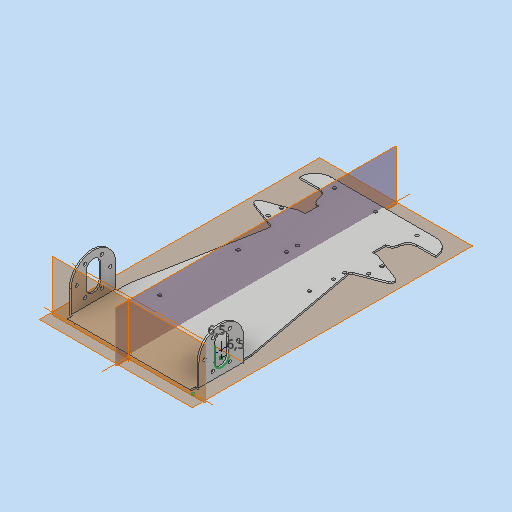
# Autodesk Inventor part: grundplatte
Saved by Autodesk Inventor 2022 (Build 260153000, 153)
## iProperties
Created: 2021-05-24
Part Number: grundplatte
Material: Generisch
Document SubType Name: Modeling
Designer: Lukas
Density: 1 g/cm^3
Appearance: Vorgabe
Author: Lukas
Autodesk Inventor part; units mm, degrees
sketch "Skizze1" plane through (0, 0, 0) normal (0, 1, 0) x (-1, 0, 0)
  line L0 (-55, 0) -> (-55, -55)
  line L1 (-55, -55) -> (-35.3027, -161.5294)
  line L2 (0, 0) -> (-55, 0)
  line L3 (79.5383, 0) -> (-92.2301, 0) projected
  line L4 (-36.5551, -163.7611) -> (-60.3632, -172.8644)
  line L5 (-60.3632, -178.4687) -> (-35, -188.1665)
  line L6 (-35, -188.1665) -> (-30, -188.1665)
  line L7 (-30, -188.1665) -> (-30, -200.1665)
  line L8 (-30, -200.1665) -> (-30, -200.1665)
  line L9 (-36, -206.1665) -> (-36, -206.1665)
  line L10 (-36, -206.1665) -> (-36, -206.1665)
  line L11 (-44, -214.1665) -> (-44, -214.1665)
  line L12 (-44, -214.1665) -> (-61, -214.1665)
  line L13 (-61, -214.1665) -> (-61, -214.1665)
  line L14 (-47, -228.1665) -> (-47, -228.1665)
  line L15 (-47, -228.1665) -> (0, -228.1665)
  arc A0 (-61, -214.1665) -> (-47, -228.1665) centre (-47, -214.1665) ccw
  arc A1 (-44, -214.1665) -> (-36, -206.1665) centre (-44, -206.1665) ccw
  arc A2 (-30, -200.1665) -> (-36, -206.1665) centre (-30, -206.1665) ccw
  arc A3 (-60.3632, -172.8644) -> (-60.3632, -178.4687) centre (-59.2917, -175.6665) ccw
  arc A4 (-36.5551, -163.7611) -> (-35.3027, -161.5294) centre (-37.2694, -161.893) ccw
  line L16 (0, 0) -> (0, -228.1665)
  point P0 (-35, -163.1665)
  point P1 (-67.6917, -175.6665)
  point P2 (-36, -200.1665)
  point P3 (-36, -214.1665)
  point P4 (-61, -228.1665)
  dimension "d1" = 55
  dimension "d54" = 110
  dimension "d55" = 55
  dimension "d56" = 20
  dimension "d57" = 35
  dimension "d58" = 35
  dimension "d59" = 25
  dimension "d60" = 12.5
  dimension "d61" = 5
  dimension "d62" = 12
  dimension "d63" = 6
  dimension "d64" = 6
  dimension "d65" = 8
  dimension "d66" = 8
  dimension "d67" = 17
  dimension "d68" = 14
  dimension "d69" = 14
  dimension "d70" = 47
  dimension "d71" = 14
  dimension "d72" = 8
  dimension "d73" = 6
  dimension "d74" = 3
  dimension "d75" = 2
  constraints: 32 end point, 14 point on line, 10 point on circle, 10 tangent, 6 perpendicular, 5 centre point, 2 vertical, 1 horizontal
  measures "d1" distance of L0.start L0.end
  measures "d54" distance of L0.end point (-35, -163.167)
  measures "d55" distance of L2.start L0.start
  measures "d56" horizontal distance of L0.end point (-35, -163.167)
  measures "d57" distance of point (-35, -163.167) point (-67.692, -175.667)
  measures "d58" distance of point (-67.692, -175.667) L5.end
  measures "d59" distance of L5.end point (-35, -163.167)
  measures "d60" vertical distance of point (-35, -163.167) point (-67.692, -175.667)
  measures "d61" distance of L5.end L6.end
  measures "d62" distance of L6.end L7.end
  measures "d63" distance of L7.end point (-36, -200.167)
  measures "d64" distance of point (-36, -200.167) L9.end
  measures "d65" distance of L9.end point (-36, -214.167)
  measures "d66" distance of point (-36, -214.167) L11.end
  measures "d67" distance of L11.end L12.end
  measures "d68" distance of L12.end point (-61, -228.167)
  measures "d69" distance of point (-61, -228.167) L14.end
  measures "d70" distance of L14.end L15.end
  measures "d71" radius of A0
  measures "d72" radius of A1
  measures "d73" radius of A2
  measures "d74" radius of A3
  measures "d75" radius of A4
extrude "Extrusion1" add sketch "Skizze1" along normal blind 1.5
mirror "Spiegeln1" about plane through (0, 0, 0) normal (1, 0, 0) of "Extrusion1"
sketch "Skizze2" plane through (0, 1.5, 0) normal (0, 1, 0) x (1, 0, 0)
  line L0 (55, 0) -> (-55, 0) projected
  line L1 (-55, 0) -> (-55, 55) projected
  line L2 (55, 0) -> (55, 55) projected
  arc A0 (60.3632, 172.8644) -> (60.3632, 178.4687) centre (59.2917, 175.6665) ccw projected
  line L3 (47, 228.1665) -> (-47, 228.1665) projected
  point P0 (0, 0)
  point P1 (-32, 60)
  point P2 (32, 60)
  point P3 (-32, 130)
  point P4 (32, 130)
  point P5 (33.5, 150)
  point P6 (33.5, 160)
  point P7 (-8.8, 160)
  point P8 (-8.8, 150)
  point P9 (45, 170)
  point P10 (45, 182)
  point P11 (0, 221.1665)
  point P12 (37, 221.1665)
  point P13 (-37, 221.1665)
  point P14 (-45, 182)
  point P15 (-45, 170)
  dimension "d78" = 60
  dimension "d79" = 23
  dimension "d80" = 60
  dimension "d81" = 23
  dimension "d82" = 70
  dimension "d83" = 70
  dimension "d84" = 23
  dimension "d85" = 23
  dimension "d86" = 20
  dimension "d87" = 1.5
  dimension "d88" = 10
  dimension "d89" = 1.5
  dimension "d91" = 20
  dimension "d92" = 10
  dimension "d93" = 42.3
  dimension "d94" = 42.3
  dimension "d95" = 13
  dimension "d97" = 10
  dimension "d98" = 13
  dimension "d99" = 12
  dimension "d100" = 7
  dimension "d101" = 7
  dimension "d102" = 7
  dimension "d103" = 10
  dimension "d104" = 37
  dimension "d105" = 37
  dimension "d106" = 10
  dimension "d107" = 12
  dimension "d108" = 40
  dimension "d109" = 13
  dimension "d110" = 13
  measures "d78" distance from line of L0 point (-32, 60)
  measures "d79" distance from line of L1 point (-32, 60)
  measures "d80" distance from line of L0 point (32, 60)
  measures "d81" distance from line of L2 point (32, 60)
  measures "d82" distance of point (-32, 60) point (-32, 130)
  measures "d83" distance of point (32, 60) point (32, 130)
  measures "d84" distance from line of L1 point (-32, 130)
  measures "d85" distance from line of L2 point (32, 130)
  measures "d86" vertical distance of point (32, 130) point (33.5, 150)
  measures "d87" horizontal distance of point (32, 130) point (33.5, 150)
  measures "d88" distance of point (33.5, 150) point (33.5, 160)
  measures "d89" horizontal distance of point (32, 130) point (33.5, 160)
  measures "d91" vertical distance of point (32, 130) point (-8.8, 150)
  measures "d92" distance of point (-8.8, 150) point (-8.8, 160)
  measures "d93" distance of point (33.5, 150) point (-8.8, 150)
  measures "d94" distance of point (33.5, 160) point (-8.8, 160)
  measures "d95" horizontal distance of point (45, 170) point (32, 130)
  measures "d97" vertical distance of point (33.5, 160) point (45, 170)
  measures "d98" horizontal distance of point (32, 130) point (45, 182)
  measures "d99" distance of point (45, 170) point (45, 182)
  measures "d100" distance from line of L3 point (37, 221.167)
  measures "d101" distance from line of L3 point (0, 221.167)
  measures "d102" distance from line of L3 point (-37, 221.167)
  measures "d103" horizontal distance of L3.start point (37, 221.167)
  measures "d104" distance of point (37, 221.167) point (0, 221.167)
  measures "d105" distance of point (0, 221.167) point (-37, 221.167)
  measures "d106" horizontal distance of L3.end point (-37, 221.167)
  measures "d107" distance of point (-45, 170) point (-45, 182)
  measures "d108" vertical distance of point (-32, 130) point (-45, 170)
  measures "d109" horizontal distance of point (-45, 170) point (-32, 130)
  measures "d110" horizontal distance of point (-32, 130) point (-45, 182)
hole "Bohrung1" at (-32, 1.5, -60) at (32, 1.5, -60) at (-32, 1.5, -130) at (32, 1.5, -130) at (33.5, 1.5, -150) at (33.5, 1.5, -160) at (-8.8, 1.5, -160) at (-8.8, 1.5, -150) at (45, 1.5, -170) at (45, 1.5, -182) at (0, 1.5, -221.1665) at (37, 1.5, -221.1665) at (-37, 1.5, -221.1665) at (-45, 1.5, -182) at (-45, 1.5, -170) direction (0, -1, 0) diameter 3 end through all
sketch "Skizze4" plane through (55, 0, 0) normal (1, 0, 0) x (0, 0, -1)
  line L0 (0, 1.5) -> (55, 1.5) projected
  line L1 (5, 1.5) -> (45, 1.5)
  line L2 (45, 1.5) -> (45, 0)
  line L3 (45, 0) -> (5, 0)
  line L4 (0, 0) -> (55, 0) projected
  line L5 (5, 1.5) -> (5, 0)
  line L6 (0, 0) -> (0, 1.5) projected
  dimension "d121" = 40
  dimension "d122" = 5
  dimension "d123" = 40
  constraints: 8 end point, 3 point on line, 2 perpendicular
  measures "d121" distance of L1.start L1.end
  measures "d122" distance between parallel lines of L6 L5
  measures "d123" distance of L2.end L3.end
extrude "Extrusion2" add sketch "Skizze4" along normal blind 3 contours L0 L2 L3 L5
sketch "Skizze5" plane through (0, 1.5, 0) normal (0, 1, 0) x (1, 0, 0)
  line L0 (55, 5) -> (58, 5) projected
  line L1 (56.5, 5) -> (56.5, 45)
  line L2 (55, 45) -> (58, 45) projected
  line L3 (58, 45) -> (58, 5)
  line L4 (58, 5) -> (56.5, 5)
  line L5 (56.5, 45) -> (58, 45)
  point P0 (0, 0)
  dimension "d126" = 1.5
  constraints: 8 end point, 2 midpoint, 1 collinear, 1 perpendicular, 1 vertical
  measures "d126" distance from line of L0.start L1
extrude "Extrusion3" add sketch "Skizze5" along normal blind 40
fillet "Rundung1" radius 2 1 edges at (58, 0, -25)
fillet "Rundung2" radius 20 2 edges at (57.25, 41.5, -5) (57.25, 41.5, -45)
mirror "Spiegeln2" about plane through (0, 0, 0) normal (1, 0, 0) of "Extrusion2", "Extrusion3"
mirror "Spiegeln3" about plane through (0, 0, 0) normal (1, 0, 0) of "Rundung2"
sketch "Skizze6" plane through (58, 0, 0) normal (1, 0, 0) x (0, 0, -1)
  arc A0 (18.5, 15) -> (31.5, 15) centre (25, 15) ccw
  arc A1 (31.5, 28.5) -> (18.5, 28.5) centre (25, 28.5) ccw
  line L0 (5, 2) -> (5, 21.5) projected
  line L1 (45, 2) -> (5, 2) projected
  line L2 (18.5, 28.5) -> (18.5, 15)
  line L3 (31.5, 28.5) -> (31.5, 15)
  line L4 (45, 1.5) -> (55, 1.5) projected
  point P0 (0, 0)
  dimension "d131" = 13
  dimension "d132" = 13
  dimension "d133" = 20
  dimension "d135" = 20
  dimension "d136" = 13.5
  dimension "d143" = 13.5
  constraints: 4 end point, 4 point on circle, 4 tangent, 2 centre point
  measures "d131" diameter of A0
  measures "d132" diameter of A1
  measures "d133" distance from line of L0 A0.centre
  measures "d135" distance from line of L0 A1.centre
  measures "d136" distance of A0.centre A1.centre
  measures "d143" distance from line of L4 A0.centre
extrude "Extrusion4" cut sketch "Skizze6" against normal blind 1.5
sketch "Skizze7" plane through (58, 0, 0) normal (1, 0, 0) x (0, 0, -1)
  line L0 (0, 1.5) -> (5, 1.5) projected
  line L1 (45, 1.5) -> (55, 1.5) projected
  line L2 (5, 2) -> (5, 21.5) projected
  line L3 (45, 2) -> (45, 21.5) projected
  line L4 (45, 2) -> (5, 2) projected
  line L5 (18.5, 15) -> (18.5, 28.5) projected
  arc A0 (18.5, 15) -> (31.5, 15) centre (25, 15) ccw projected
  point P0 (0, 0)
  point P1 (10, 21.5)
  dimension "d146" = 20
  dimension "d147" = 5
  measures "d146" distance from line of L0 point (10, 21.5)
  measures "d147" distance from line of L2 point (10, 21.5)
sketch "Skizze8" plane through (58, 0, 0) normal (1, 0, 0) x (0, 0, -1)
  line L0 (18.5, 15) -> (18.5, 28.5) projected
  arc A0 (18.5, 15) -> (31.5, 15) centre (25, 15) ccw projected
  point P0 (0, 0)
  point P1 (25, 21.5)
  dimension "d150" = 6.5
  dimension "d151" = 6.5
  measures "d150" distance from line of L0 point (25, 21.5)
  measures "d151" distance of A0.centre point (25, 21.5)
hole "Bohrung2" at (58, 21.5, -10) direction (-1, 0, 0) diameter 3 end through all
pattern_circular "Runde Anordnung1" count 6 over 360 about axis through (58, 21.5, -25) along (1, 0, 0) of "Bohrung2"
mirror "Spiegeln4" about plane through (0, 0, 0) normal (1, 0, 0) of "Extrusion4"
ref_plane "Arbeitsebene1" through (0, 0, 0) normal (1, 0, 0) x (0, 1, 0)
